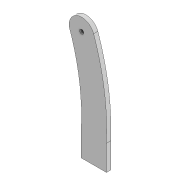
# Autodesk Inventor part: Stütze vorne
Saved by Autodesk Inventor 2020 (Build 240168000, 168)
## iProperties
Created: 2021-06-23
Part Number: Stütze vorne
Material: Generisch
Document SubType Name: Modeling
Designer: mike8
Density: 1 g/cm^3
Appearance: Vorgabe
Author: mike8
Autodesk Inventor part; units mm, degrees
ref_plane "YZ Plane" through (0, 0, 0) normal (1, 0, 0) x (0, 1, 0)
ref_plane "XZ Plane" through (0, 0, 0) normal (0, 1, 0) x (-1, 0, 0)
ref_plane "XY Plane" through (0, 0, 0) normal (0, 0, 1) x (1, 0, 0)
sketch "Skizze1" plane through (0, 0, 0) normal (0, 0, 1) x (1, 0, 0)
  line L0 (-319.4908, 0) -> (79.1023, 0) projected
  line L1 (0, -57.6247) -> (0, 149.9482) projected
  line L2 (17.1489, -27.9715) -> (-12.8511, -27.9715)
  line L3 (-12.8511, -27.9715) -> (-12.8511, 2.0285)
  line L4 (-12.8511, 2.0285) -> (17.1489, 2.0285)
  line L5 (17.1489, 2.0285) -> (17.1489, -27.9715)
  arc A0 (1.933, 106.9528) -> (-27.0148, 99.4639) centre (-12.2357, 102.0285) ccw
  arc A1 (-12.8511, 2.0285) -> (-27.0148, 99.4639) centre (-262.4886, 15.487) ccw
  arc A2 (17.1489, 2.0285) -> (1.933, 106.9528) centre (-262.5489, 15.0327) ccw
  point P0 (0, 0)
  dimension "d0" = 30
  dimension "d1" = 30
  dimension "d2" = 30
  dimension "d4" = 100
  dimension "d6" = 250
  dimension "d7" = 280
  constraints: 8 end point, 6 point on circle, 3 centre point, 2 parallel, 1 horizontal, 1 perpendicular, 1 tangent
  measures "d0" distance of L2.start L2.end
  measures "d1" distance of L4.end L2.start
  measures "d2" diameter of A0
  measures "d4" distance from line of A0.centre L4
  measures "d6" radius of A1
  measures "d7" radius of A2
extrude "Extrusion1" add sketch "Skizze1" along normal blind 5
sketch "Skizze2" plane through (0, 0, 5) normal (0, 0, 1) x (1, 0, 0)
  arc A0 (1.933, 106.9528) -> (-27.0148, 99.4639) centre (-12.2357, 102.0285) ccw projected
  point P0 (0, 0)
  dimension "d10" = 0
  dimension "d11" = 0
  measures "d10" distance of A0.centre point (-12.236, 102.029)
  measures "d11" distance of A0.centre point (-12.236, 102.029)
hole "Bohrung1" at (-12.2357, 102.0285, 5) direction (0, 0, -1) diameter 5 end through all
